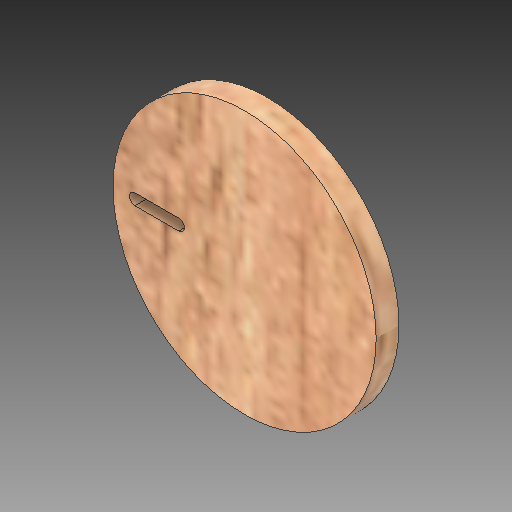
# Autodesk Inventor part: KnobCover
Saved by Autodesk Inventor 2018 (Build 220112000, 112)
## iProperties
Created: 2017-12-06
Part Number: KnobCover
Material: Wood (Birch)
Document SubType Name: Modeling
Designer: Andrew
Density: 0.55 g/cm^3
Appearance: Birch - Natural Polished
Author: Andrew
Autodesk Inventor part; units mm, degrees
ref_plane "YZ Plane" through (0, 0, 0) normal (1, 0, 0) x (0, 1, 0)
ref_plane "XZ Plane" through (0, 0, 0) normal (0, 1, 0) x (-1, 0, 0)
ref_plane "XY Plane" through (0, 0, 0) normal (0, 0, 1) x (1, 0, 0)
sketch "Sketch1" plane through (0, 0, 0) normal (0, 0, 1) x (1, 0, 0)
  circle A0 centre (0, 0) radius 19.05
  line L0 (-15.875, 0) -> (-9.525, 0) construction
  line L1 (-15.875, 0.8128) -> (-9.525, 0.8128)
  line L2 (-9.525, -0.8128) -> (-15.875, -0.8128)
  arc A1 (-15.875, 0.8128) -> (-15.875, -0.8128) centre (-15.875, 0) ccw
  arc A2 (-9.525, -0.8128) -> (-9.525, 0.8128) centre (-9.525, 0) ccw
  point P0 (-12.7, 0)
  dimension "d0" = 38.1
  dimension "d1" = 6.35
  dimension "d2" = 12.7
  dimension "d3" = 1.6256
  constraints: 8 end point, 4 point on circle, 4 tangent, 3 centre point, 1 coincident, 1 horizontal, 1 midpoint, 1 parallel, 1 point on line
  measures "d0" diameter of A0
  measures "d1" distance of L0.start L0.end
  measures "d2" distance of point (-12.7, 0) point (0, 0)
  measures "d3" distance between parallel lines of L2 L1
derived "Knob.ipt"
derived "Enclosure Top.ipt"
extrude "Extrusion1" add sketch "Sketch1" along normal blind 3.302
equation "\"d6\" = encThick"
equation "\"encThick\" = 3.302"
body "Solid1"
